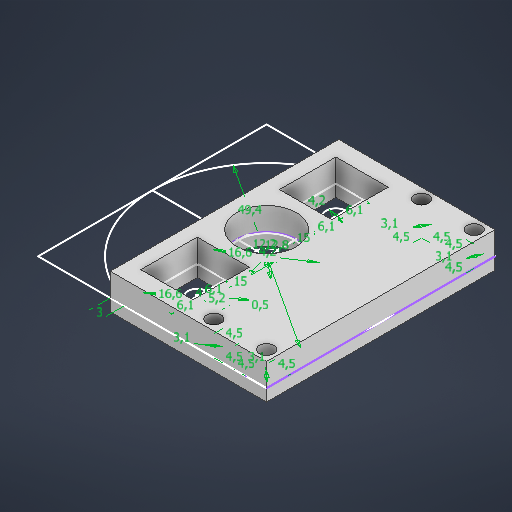
# Autodesk Inventor part: peça1
Saved by Autodesk Inventor 2026 (Build 300175000, 175)
## iProperties
Created: 2026-04-17
Part Number: peça1
Material: Genérico
Document SubType Name: Modeling
Designer: a2453266
Density: 1 g/cm^3
Appearance: Padrão
Author: a2453266
## iProperties of the stored document peça1_3DPrint.ipt
Created: 2026-04-17
Part Number: peça1_3DPrint
Material: Genérico
Document SubType Name: Modeling
Designer: a2453266
Density: 1 g/cm^3
Appearance: Padrão
Author: a2453266
Autodesk Inventor part; units mm, degrees
ref_plane "YZ Plane" through (0, 0, 0) normal (1, 0, 0) x (0, 1, 0)
ref_plane "XZ Plane" through (0, 0, 0) normal (0, 1, 0) x (-1, 0, 0)
ref_plane "XY Plane" through (0, 0, 0) normal (0, 0, 1) x (1, 0, 0)
sketch "Esboço1" plane through (0, 0, 0) normal (0, 1, 0) x (-1, 0, 0)
  circle A0 centre (0, 0) radius 2.1
  line L0 (0, 0) -> (0, 15)
  circle A1 centre (0, 15) radius 2
  line L1 (0, 0) -> (0, -15)
  circle A2 centre (0, -15) radius 2.1
  line L2 (0, 15) -> (-5.2, 15)
  line L3 (-5.2, 15) -> (-5.2, -15)
  line L4 (-5.2, -15) -> (0, -15)
  circle A3 centre (0, 0) radius 6.1
  circle A4 centre (0, 0) radius 24.7
  line L5 (0, 24.7) -> (24.7, 24.7)
  line L6 (24.7, 24.7) -> (24.7, 0)
  line L7 (24.7, 0) -> (0, 0)
  line L8 (0, 0) -> (0, 24.7)
  line L9 (24.7, 0) -> (0, 0)
  line L10 (0, 0) -> (0, -24.7)
  line L11 (0, -24.7) -> (24.7, -24.7)
  line L12 (24.7, -24.7) -> (24.7, 0)
  line L13 (0, -24.7) -> (-24.7, -24.7)
  line L14 (-24.7, -24.7) -> (-24.7, 0)
  line L15 (-24.7, 0) -> (0, 0)
  line L16 (0, 0) -> (0, -24.7)
  line L17 (0, 24.7) -> (-24.7, 24.7)
  line L18 (-24.7, 24.7) -> (-24.7, 0)
  line L19 (-24.7, 0) -> (0, 0)
  line L20 (0, 0) -> (0, 24.7)
  line L21 (-5.2, 15) -> (-5.2, 24.7)
  line L22 (-5.2, -15) -> (-5.2, -24.7)
  line L23 (-5.2, 24.7) -> (-24.7, 24.7)
  line L24 (-24.7, 24.7) -> (-24.7, -24.7)
  line L25 (-24.7, -24.7) -> (-5.2, -24.7)
  line L26 (-5.2, -24.7) -> (-5.2, 24.7)
  line L27 (0, -15) -> (0, -21.1)
  line L28 (0, -21.1) -> (-5.2, -21.1)
  line L29 (0, -15) -> (0, -8.9)
  line L30 (0, -8.9) -> (-5.2, -8.9)
  line L31 (0, -8.9) -> (0, -15)
  line L32 (0, 15) -> (0, 8.9)
  line L33 (0, 15) -> (0, 21.1)
  line L34 (0, 21.1) -> (-5.2, 21.1)
  line L35 (0, 8.9) -> (-5.2, 8.9)
  line L36 (6.1, 0) -> (6.1, -24.7)
  line L37 (6.1, 0) -> (6.1, 24.7)
  line L38 (-5.2, 21.1) -> (6.1, 21.1)
  line L39 (6.1, 21.1) -> (6.1, 24.7)
  line L40 (6.1, 24.7) -> (-5.2, 24.7)
  line L41 (-5.2, 24.7) -> (-5.2, 21.1)
  line L42 (-5.2, -21.1) -> (6.1, -21.1)
  line L43 (6.1, -21.1) -> (6.1, -24.7)
  line L44 (6.1, -24.7) -> (-5.2, -24.7)
  line L45 (-5.2, -24.7) -> (-5.2, -21.1)
  line L46 (6.1, 21.1) -> (0, 21.1)
  line L47 (0, 21.1) -> (0, 8.9)
  line L48 (0, 8.9) -> (6.1, 8.9)
  line L49 (6.1, 8.9) -> (6.1, 21.1)
  line L50 (0, -8.9) -> (6.1, -8.9)
  line L51 (6.1, -8.9) -> (6.1, -21.1)
  line L52 (6.1, -21.1) -> (0, -21.1)
  line L53 (0, -21.1) -> (0, -8.9)
  line L54 (6.1, -24.7) -> (9.1, -24.7)
  line L55 (9.1, -24.7) -> (9.1, 24.7)
  line L56 (9.1, 24.7) -> (6.1, 24.7)
  line L57 (6.1, 24.7) -> (6.1, -24.7)
  circle A5 centre (0, 0) radius 8.3
  circle A6 centre (0, 15) radius 8.3
  line L58 (-5.2, -8.9) -> (-24.7, -8.9)
  line L59 (-24.7, -8.9) -> (-24.7, -24.7)
  line L60 (-24.7, -24.7) -> (-5.2, -24.7)
  line L61 (-5.2, -24.7) -> (-5.2, -8.9)
  line L62 (-5.2, 8.9) -> (-24.7, 8.9)
  line L63 (-24.7, 8.9) -> (-24.7, 24.7)
  line L64 (-24.7, 24.7) -> (-5.2, 24.7)
  line L65 (-5.2, 24.7) -> (-5.2, 8.9)
  line L66 (-8.3, 0) -> (-8.3, -8.9)
  line L67 (-8.3, 0) -> (-8.3, 8.9)
  line L68 (-8.3, -8.9) -> (-8.8, -8.9)
  line L69 (-8.8, -8.9) -> (-8.8, 8.9)
  line L70 (-8.8, 8.9) -> (-8.3, 8.9)
  line L71 (-8.3, 8.9) -> (-8.3, -8.9)
  line L72 (-8.8, -8.9) -> (-24.7, -8.9)
  line L73 (-24.7, -8.9) -> (-24.7, -24.7)
  line L74 (-24.7, -24.7) -> (-8.8, -24.7)
  line L75 (-8.8, -24.7) -> (-8.8, -8.9)
  line L76 (-8.8, -8.9) -> (-24.7, -8.9)
  line L77 (-24.7, -8.9) -> (-24.7, 24.7)
  line L78 (-24.7, 24.7) -> (-8.8, 24.7)
  line L79 (-8.8, 24.7) -> (-8.8, -8.9)
  line L80 (9.1, -24.7) -> (6.1, -24.7)
  line L81 (6.1, -24.7) -> (6.1, -21.1)
  line L82 (6.1, -21.1) -> (9.1, -21.1)
  line L83 (9.1, -21.1) -> (9.1, -24.7)
  line L84 (6.1, 21.1) -> (9.1, 21.1)
  line L85 (9.1, 21.1) -> (9.1, 24.7)
  line L86 (9.1, 24.7) -> (6.1, 24.7)
  line L87 (6.1, 24.7) -> (6.1, 21.1)
  line L88 (9.1, 24.7) -> (9.1, 22.9)
  line L89 (-24.7, -24.7) -> (-21.7, -24.7)
  line L90 (-24.7, -21.1) -> (-24.7, -24.7)
  line L91 (-24.7, 24.7) -> (-21.7, 24.7)
  line L92 (-24.7, 21.1) -> (-24.7, 24.7)
  line L93 (-24.7, -24.7) -> (-20.2, -24.7)
  line L94 (-20.2, -24.7) -> (-20.2, -20.2)
  line L95 (-20.2, -20.2) -> (-24.7, -20.2)
  line L96 (-24.7, -20.2) -> (-24.7, -24.7)
  line L97 (-24.7, 24.7) -> (-20.2, 24.7)
  line L98 (-20.2, 24.7) -> (-20.2, 20.2)
  line L99 (-20.2, 20.2) -> (-24.7, 20.2)
  line L100 (-24.7, 20.2) -> (-24.7, 24.7)
  line L101 (-8.8, -24.7) -> (-13.3, -24.7)
  line L102 (-13.3, -24.7) -> (-13.3, -20.2)
  line L103 (-13.3, -20.2) -> (-8.8, -20.2)
  line L104 (-8.8, -20.2) -> (-8.8, -24.7)
  line L105 (-8.8, 24.7) -> (-13.3, 24.7)
  line L106 (-13.3, 24.7) -> (-13.3, 20.2)
  line L107 (-13.3, 20.2) -> (-8.8, 20.2)
  line L108 (-8.8, 20.2) -> (-8.8, 24.7)
  line L109 (-13.3, -22.45) -> (-8.8, -22.45)
  line L110 (-20.2, -22.45) -> (-24.7, -22.45)
  line L111 (-20.2, 22.45) -> (-24.7, 22.45)
  line L112 (-8.8, 22.45) -> (-13.3, 22.45)
  circle A7 centre (-11.05, -22.45) radius 1.55
  circle A8 centre (-22.45, -22.45) radius 1.55
  circle A9 centre (-11.05, 22.45) radius 1.55
  circle A10 centre (-22.45, 22.45) radius 1.55
  circle A11 centre (0, 0) radius 6.4
  point P0 (-5.2, -3.189)
  point P1 (-5.2, 3.189)
  point P2 (-5.2, 24.1464)
  point P3 (-5.2, -24.1464)
  point P4 (6.1, -21.1)
  point P5 (6.1, 21.1)
  dimension "d6" = 12.2
  dimension "d19" = 16.6
  dimension "d0" = 4.2
  dimension "d1" = 15
  dimension "d2" = 4
  dimension "d3" = 15
  dimension "d4" = 4.2
  dimension "d5" = 5.2
  dimension "d7" = 49.4
  dimension "d8" = 6.1
  dimension "d9" = 6.1
  dimension "d10" = 6.1
  dimension "d11" = 6.1
  dimension "d16" = 3
  dimension "d20" = 16.6
  dimension "d21" = 0.5
  dimension "d29" = 4.5
  dimension "d30" = 4.5
  dimension "d31" = 4.5
  dimension "d32" = 4.5
  dimension "d33" = 4.5
  dimension "d34" = 4.5
  dimension "d35" = 4.5
  dimension "d36" = 4.5
  dimension "d37" = 3.1
  dimension "d38" = 3.1
  dimension "d39" = 3.1
  dimension "d40" = 3.1
  dimension "d45" = 12.8
  constraints: 226 end point, 43 parallel, 31 perpendicular, 24 horizontal, 21 point on line, 13 midpoint, 10 centre point, 8 coincident, 4 point on circle, 4 vertical, 1 horizontal alignment, 5 other
  measures "d0" diameter of A0
  measures "d1" distance of L0.start L0.end
  measures "d2" diameter of A1
  measures "d3" distance of L0.start L1.end
  measures "d4" diameter of A2
  measures "d5" distance of L2.start L2.end
  measures "d7" diameter of A4
  measures "d8" distance of L4.end L27.end
  measures "d9" distance of L4.end L29.end
  measures "d10" distance of L2.start L32.end
  measures "d11" distance of L2.start L33.end
  measures "d16" distance of L56.end L55.end
  measures "d20" diameter of A6
  measures "d21" distance of L69.end L70.end
  measures "d29" distance of L95.end L94.end
  measures "d30" distance of L94.end L93.end
  measures "d31" distance of L98.end L99.end
  measures "d32" distance of L97.end L98.end
  measures "d33" distance of L102.end L103.end
  measures "d34" distance of L101.end L102.end
  measures "d35" distance of L107.end L106.end
  measures "d36" distance of L106.end L105.end
  measures "d37" diameter of A7
  measures "d38" diameter of A8
  measures "d39" diameter of A9
  measures "d40" diameter of A10
  measures "d45" diameter of A11
extrude "Extrusão1" add sketch "Esboço1" along normal blind 5 contours A3 L15 A11 L3 | L3 A11 L15 A3 | A11 L15 A5 L3 | L3 A5 L15 A11 | A5 L67 L62 A6 L3 | L3 L58 L66 A5 | L66 L58 L69 L15 | L15 L69 L62 L67 | A6 L62 L3 | L3 L22 A4 L75 L58 | L69 L58 A4 L15 | L15 A4 L62 L69 | L62 L79 A4 L21 A6 | L62 A6 L21 L3 | L75 L103 L102 A4 L58 | L62 A4 L106 L107 L79 | L75 L109 A7 A4 L102 L103 | L107 L106 A4 A9 L112 L79 | A4 A7 L109 L75 | L112 A9 A4 L79 | A4 L109 A7 | A4 L112 A9 | A7 L109 A4 | L112 A4 A9 picked at (-9.9489, -22.4881) picked at (-11.1489, 21.6171) picked at (-11.1489, -21.6171) picked at (-9.9489, 22.4881)
extrude "Extrusão2" add sketch "Esboço1" along normal blind 5 contours L36 A11 L1 A3 | A3 L0 A11 L37 | A3 L3 A11 L0 | L1 A11 L3 A3 | L36 A5 L1 A11 | A11 L0 A6 A5 L37 | A11 L3 A5 A6 L0 | L1 A5 L3 A11 | L36 L50 L1 A5 | A5 A6 L48 L37 | A6 A5 L0 | L0 A5 A6 | L1 L30 L3 A5 | A5 L0 L48 A6 | A5 A6 L3 L35 L0 | A5 L3 A6 | L36 A4 L10 L42 | L38 A6 L8 A4 L37 | L36 L11 A4 | L10 A4 L22 L28 | A4 L5 L37 | L38 L8 A6 | L13 L22 A4 | L18 L62 A4 | A4 L58 L14 | A6 L8 L34 L21 | L21 A4 L8 A6 | A4 L21 L17 | L22 L13 L75 A4 | L62 L18 L99 L98 L17 L106 A4 | A4 L102 L13 L94 L95 L14 L58 | A4 L79 L17 L21 | L75 L13 L102 L109 A7 A4 | L106 L112 A9 A4 | A4 A7 L109 L102 | L95 L94 L110 A8 L14 | L18 L111 A10 L98 L99 | A4 A9 L112 L106 L17 L79 | A7 L109 A4 | A9 L112 A4 | A4 L109 A7 | A4 L112 A9 | L13 L14 L110 A8 L94 | L18 L17 L98 L111 A10 | A8 L110 | L110 A8 | A10 L111 | L111 A10 picked at (-11.818, -22.5746) picked at (-11.7193, 22.131) picked at (-11.7193, -22.131) picked at (-11.818, 22.5746)
extrude "Extrusão3" add sketch "Esboço1" along normal blind 5 contours L37 A11 L7 | L7 A11 L36 | A11 L37 A5 L7 | L7 A5 L36 A11 | A5 L37 A6 L84 L55 L7 | L7 L55 L82 L36 A5 | L55 A4 L36 L82 | L84 L37 A4 L55 | L37 A6 | A4 L37 L5 L55 | L55 L11 L36 A4
extrude "Extrusão4" cut sketch "Esboço1" along normal through all contours A7 L109 A4 | A4 L109 A7 | A9 L112 A4 | A4 L112 A9 | A7 L109 A4 | A4 L109 A7 | L112 A4 A9 | A4 L112 A9 | A8 L110 | L110 A8 | A10 L111 | L111 A10
extrude "Extrusão5" add sketch "Esboço1" against normal blind 2.6 contours L36 A11 L1 A3 | L37 A11 L7 | L7 A11 L36 | A3 L0 A11 L37 | A3 L3 A11 L0 | L1 A11 L3 A3 | A11 L37 A5 L7 | L7 A5 L36 A11 | L36 A5 L1 A11 | A11 L0 A6 A5 L37 | A11 L3 A5 A6 L0 | A3 L15 A11 L3 | L1 A5 L3 A11 | L3 A11 L15 A3 | A5 L37 A6 L84 L55 L7 | L7 L55 L82 L36 A5 | L36 L50 L1 A5 | A5 A6 L48 L37 | A6 A5 L0 | L0 A5 A6 | A11 L15 A5 L3 | L1 L30 L3 A5 | L3 A5 L15 A11 | A5 L0 L48 A6 | A5 A6 L3 L35 L0 | A5 L3 A6 | A5 L67 L62 A6 L3 | L3 L58 L66 A5 | L55 A4 L36 L82 | L84 L37 A4 L55 | L36 A4 L10 L42 | L37 A6 | L66 L58 L69 L15 | L15 L69 L62 L67 | A6 L62 L3 | L3 L22 A4 L75 L58 | A4 L37 L5 L55 | L55 L11 L36 A4 | L38 A6 L8 A4 L37 | L36 L11 A4 | L10 A4 L22 L28 | L69 L58 A4 L15 | L15 A4 L62 L69 | L62 L79 A4 L21 A6 | L62 A6 L21 L3 | A4 L5 L37 | L38 L8 A6 | L13 L22 A4 | L18 L62 A4 | A4 L58 L14 | L75 L103 L102 A4 L58 | L62 A4 L106 L107 L79 | A6 L8 L34 L21 | L21 A4 L8 A6 | A4 L21 L17 | L22 L13 L75 A4 | L62 L18 L99 L98 L17 L106 A4 | A4 L102 L13 L94 L95 L14 L58 | L75 L109 A7 A4 L102 L103 | L107 L106 A4 A9 L112 L79 | A4 L79 L17 L21 | L75 L13 L102 L109 A7 A4 | A4 A7 L109 L75 | L106 L112 A9 A4 | A4 A7 L109 L102 | L95 L94 L110 A8 L14 | L18 L111 A10 L98 L99 | L112 A9 A4 L79 | A4 A9 L112 L106 L17 L79 | L13 L14 L110 A8 L94 | L18 L17 L98 L111 A10
extrude "Extrusão6" cut sketch "Esboço1" against normal blind 2.6 contours L7 L0 A0 | L7 A3 L1 A0 | A0 L0 A3 L7 | A0 L1 L7 | L0 L15 A0 | A0 L15 L3 A3 L0 | L1 A3 L3 L15 A0 | A0 L15 L1 | L36 A11 L1 A3 | L37 A11 L7 | L7 A11 L36 | A3 L0 A11 L37 | A3 L3 A11 L0 | L1 A11 L3 A3 | L15 A3 L3 | L3 A3 L15 | A3 L15 A11 L3 | L3 A11 L15 A3
extrude "Extrusão7" cut sketch "Esboço1" along normal through all contours L7 L0 A0 | L7 A3 L1 A0 | A0 L0 A3 L7 | A0 L1 L7 | L0 L15 A0 | A0 L15 L3 A3 L0 | L1 A3 L3 L15 A0 | A0 L15 L1 | L36 A11 L1 A3 | L37 A11 L7 | L7 A11 L36 | A3 L0 A11 L37 | A3 L3 A11 L0 | L1 A11 L3 A3 | L15 A3 L3 | L3 A3 L15 | A3 L15 A11 L3 | L3 A11 L15 A3
